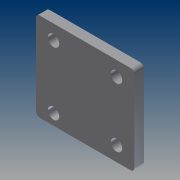
# Autodesk Inventor part: MotorMountBottom
Saved by Autodesk Inventor 2011 SP1 (Build 150282100, 282)
## iProperties
Created: 2011-07-18
Part Number: MotorMountBottom
Document SubType Name: Modeling
Designer: Nathan
Density: 1 g/cm^3
Author: Nathan
Autodesk Inventor part; units mm, degrees
ref_plane "YZ Plane" through (0, 0, 0) normal (1, 0, 0) x (0, 1, 0)
ref_plane "XZ Plane" through (0, 0, 0) normal (0, 1, 0) x (-1, 0, 0)
ref_plane "XY Plane" through (0, 0, 0) normal (0, 0, 1) x (1, 0, 0)
sketch "Sketch1" plane through (0, 0, 0) normal (0, 0, 1) x (1, 0, 0)
  line L0 (-15.875, -14.2875) -> (15.875, -14.2875)
  line L1 (15.875, -14.2875) -> (15.875, 14.2875)
  line L2 (15.875, 14.2875) -> (-15.875, 14.2875)
  line L3 (-15.875, 14.2875) -> (-15.875, -14.2875)
  line L4 (0, 0) -> (0, 6.6196)
  line L5 (-8.6733, 0) -> (9.2317, 0)
  circle A0 centre (-10.16, 9.525) radius 1.8288
  circle A1 centre (10.16, 9.525) radius 1.8288
  circle A2 centre (10.16, -9.525) radius 1.8288
  circle A3 centre (-10.16, -10.795) radius 1.8288
  dimension "d3" = 31.75
  dimension "d4" = 28.575
  dimension "d27" = 20.32
  dimension "d28" = 10.16
  dimension "d29" = 3.6576
  dimension "d30" = 3.6576
  dimension "d31" = 3.6576
  dimension "d32" = 3.6576
  constraints: 12 end point, 4 centre point, 4 coincident, 3 parallel, 2 horizontal, 2 perpendicular, 1 vertical, 2 other
  measures "d3" distance of L2.end L1.end
  measures "d4" distance of L1.end L0.end
  measures "d27" distance of point (-10.16, 9.525) point (-10.16, -10.795)
  measures "d28" distance from line of L4 point (-10.16, 9.525)
  measures "d29" diameter of A0
  measures "d30" diameter of A1
  measures "d31" diameter of A2
  measures "d32" diameter of A3
extrude "Extrusion1" add sketch "Sketch1" along normal blind 3.175 contours L3 L2 L1 L0 | A0 | A1 | A2 | A3
fillet "Fillet1" radius 1.27 1 edges at (15.875, 14.2875, 1.5875)
fillet "Fillet2" radius 1.27 1 edges at (-15.875, 14.2875, 1.5875)
fillet "Fillet3" radius 1.27 1 edges at (15.875, -14.2875, 1.5875)
fillet "Fillet4" radius 1.27 1 edges at (-15.875, -14.2875, 1.5875)
extrude "Extrusion2" cut sketch "Sketch1" along normal through all contours A0 | A1 | A2 | A3
body "Solid1"
